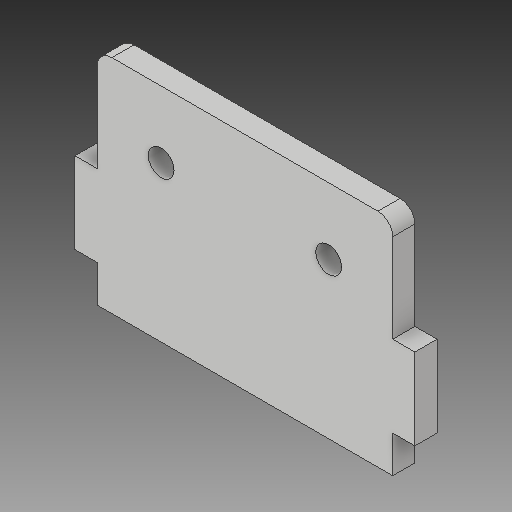
# Autodesk Inventor part: Tope riel final
Saved by Autodesk Inventor 2019 (Build 230136000, 136)
## iProperties
Created: 2020-02-01
Part Number: Tope riel final
Material: Generic
Document SubType Name: Modeling
Designer: Elías Sánchez
Density: 1 g/cm^3
Appearance: Default
Description: Corte Láser
Author: Elías Sánchez
Autodesk Inventor part; units mm, degrees
ref_plane "YZ Plane" through (0, 0, 0) normal (1, 0, 0) x (0, 1, 0)
ref_plane "XZ Plane" through (0, 0, 0) normal (0, 1, 0) x (-1, 0, 0)
ref_plane "XY Plane" through (0, 0, 0) normal (0, 0, 1) x (1, 0, 0)
sketch "Sketch1" plane through (0, 0, 0) normal (0, 0, 1) x (1, 0, 0)
  line L0 (-40, 0) -> (40, 0)
  circle A0 centre (-22.665, 42) radius 3.5
  circle A1 centre (22.665, 42) radius 3.5
  line L1 (-40, 10) -> (-40, 0)
  line L2 (40, 60) -> (40, 32)
  line L3 (40, 32) -> (46, 32)
  line L4 (46, 32) -> (46, 10)
  line L5 (46, 10) -> (40, 10)
  line L6 (40, 10) -> (40, 0)
  line L7 (-40, 10) -> (-46, 10)
  line L8 (-46, 10) -> (-46, 32)
  line L9 (-46, 32) -> (-40, 32)
  line L10 (-40, 32) -> (-40, 60)
  line L11 (-40, 60) -> (40, 60)
  point P0 (0, 0)
  point P1 (0, 42)
  point P2 (0, 0)
  dimension "d1" = 60
  dimension "d4" = 80
  dimension "d5" = 7
  dimension "d7" = 7
  dimension "d9" = 22.665
  dimension "d10" = 22.665
  dimension "d11" = 42
  dimension "d32" = 6
  dimension "d33" = 28
  dimension "d34" = 10
  dimension "d35" = 10
  dimension "d36" = 28
  dimension "d37" = 6
  dimension "d38" = 6
  dimension "d39" = 22
  constraints: 24 end point, 8 perpendicular, 2 centre point, 2 coincident, 2 horizontal, 1 horizontal alignment, 1 midpoint, 1 point on line, 1 vertical, 1 vertical alignment
  measures "d1" distance of L0.end L2.start
  measures "d4" distance of L0.start L0.end
  measures "d5" diameter of A0
  measures "d7" diameter of A1
  measures "d9" horizontal distance of point (0, 0) A1.centre
  measures "d10" horizontal distance of point (0, 0) A0.centre
  measures "d11" distance from line of L0 A1.centre
  measures "d32" distance of L2.end L3.end
  measures "d33" distance of L2.start L2.end
  measures "d34" distance of L5.end L0.end
  measures "d35" distance of L1.start L0.start
  measures "d36" distance of L9.end L10.end
  measures "d37" distance of L8.end L9.end
  measures "d38" distance of L1.start L7.end
  measures "d39" distance of L7.end L8.end
extrude "Extrusion2" add sketch "Sketch1" along normal blind 6
fillet "Fillet3" radius 4 2 edges at (-40, 60, 3) (40, 60, 3)
equation "\"d1\" = d0"
equation "\"d7\" = d5"
equation "\"d10\" = d9"
equation "\"d32\" = d28"
equation "\"d33\" = d29"
equation "\"d35\" = d34"
equation "\"d36\" = d33"
equation "\"d37\" = d32"
equation "\"d0\" = 60"
equation "\"d28\" = 6"
equation "\"d29\" = 28"
body "Solid2"
